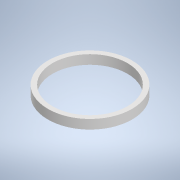
# Autodesk Inventor part: Упор
Saved by Autodesk Inventor 2021 (Build 250183000, 183)
## iProperties
Created: 2024-03-30
Part Number: Упор
Material: Типовые
Document SubType Name: Modeling
Designer: Мария
Density: 1 g/cm^3
Appearance: По умолчанию
Author: Мария
Autodesk Inventor part; units mm, degrees
ref_plane "YZ Plane" through (0, 0, 0) normal (1, 0, 0) x (0, 1, 0)
ref_plane "XZ Plane" through (0, 0, 0) normal (0, 1, 0) x (-1, 0, 0)
ref_plane "XY Plane" through (0, 0, 0) normal (0, 0, 1) x (1, 0, 0)
sketch "Эскиз1" plane through (0, 0, 0) normal (0, 0, 1) x (1, 0, 0)
  line L0 (6.5, 0) -> (6.5, 1.6)
  line L1 (6.5, 1.6) -> (7.3, 1.6)
  line L2 (7.3, 1.6) -> (7.3, 0.8)
  line L3 (7.3, 0.8) -> (7.3, 0.8)
  line L4 (7.3, 0.8) -> (7.3, 0)
  line L5 (7.3, 0) -> (6.5, 0)
  line L6 (0, 0) -> (0, 10)
  dimension "d0" = 10
  dimension "d1" = 13
  dimension "d2" = 0.8
  dimension "d3" = 0.8
  dimension "d4" = 0.8
  dimension "d5" = 1.6
  constraints: 14 end point, 4 perpendicular, 2 vertical, 1 horizontal alignment
  measures "d0" distance of L6.start L6.end
  measures "d1" diameter of L0 L6
  measures "d2" distance between parallel lines of L0 L4
  measures "d3" distance between parallel lines of L1 L3
  measures "d4" distance of L0.end L1.end
  measures "d5" distance from line of L0.start L1
revolve "Вращение1" add sketch "Эскиз1" angle 360 about axis through (0, 0, 0) along (0, 1, 0)
